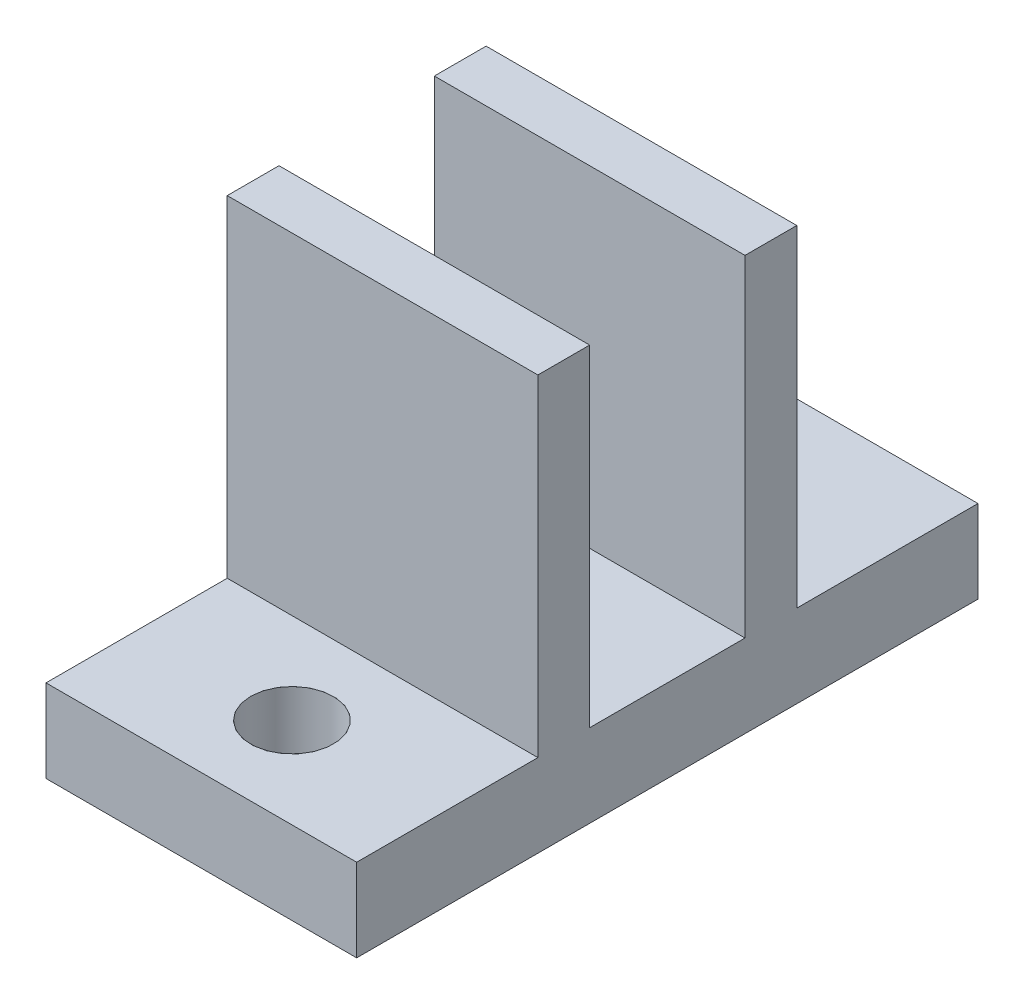
# Autodesk Inventor part: XPulleySupport
Saved by Autodesk Inventor 2019 (Build 230136000, 136)
## iProperties
Created: 2019-08-19
Part Number: XPulleySupport
Material: Generic
Document SubType Name: Modeling
Designer: Bruno
Density: 1 g/cm^3
Appearance: Default
Author: Bruno
Autodesk Inventor part; units mm, degrees
ref_plane "YZ Plane" through (0, 0, 0) normal (1, 0, 0) x (0, 1, 0)
ref_plane "XZ Plane" through (0, 0, 0) normal (0, 1, 0) x (-1, 0, 0)
ref_plane "XY Plane" through (0, 0, 0) normal (0, 0, 1) x (1, 0, 0)
sketch "Sketch1" plane through (0, 0, 0) normal (0, 1, 0) x (-1, 0, 0)
  line L0 (42.7623, -5.5692) -> (12.7623, -5.5692)
  line L1 (12.7623, 54.4308) -> (42.7623, 54.4308)
  line L2 (42.7623, 31.9308) -> (12.7623, 31.9308)
  line L3 (12.7623, 16.9308) -> (42.7623, 16.9308)
  line L4 (42.7623, 16.9308) -> (42.7623, 11.9308)
  line L5 (42.7623, 11.9308) -> (12.7623, 11.9308)
  line L6 (12.7623, 11.9308) -> (12.7623, 16.9308)
  line L7 (42.7623, 31.9308) -> (42.7623, 36.9308)
  line L8 (42.7623, 36.9308) -> (12.7623, 36.9308)
  line L9 (12.7623, 36.9308) -> (12.7623, 31.9308)
  line L10 (42.7623, 11.9308) -> (42.7623, -5.5692)
  line L11 (12.7623, 11.9308) -> (12.7623, -5.5692)
  line L12 (12.7623, 16.9308) -> (12.7623, 31.9308)
  line L13 (42.7623, 31.9308) -> (42.7623, 16.9308)
  line L14 (42.7623, 36.9308) -> (42.7623, 54.4308)
  line L15 (12.7623, 54.4308) -> (12.7623, 36.9308)
  circle A0 centre (27.7623, 3.1808) radius 4
  circle A1 centre (27.7623, 45.6808) radius 4
  line L16 (27.7623, 3.1808) -> (42.7623, 3.1808) construction
  line L17 (27.7623, 3.1808) -> (27.7623, 11.9308) construction
  line L18 (27.7623, 45.6808) -> (27.7623, 36.9308) construction
  line L19 (27.7623, 45.6808) -> (42.7623, 45.6808) construction
  point P0 (0, 0)
  dimension "d0" = 60
  dimension "d1" = 30
  dimension "d2" = 5
  dimension "d3" = 15
  dimension "d4" = 8
  dimension "d5" = 8
  constraints: 40 end point, 5 equal length, 5 perpendicular, 4 midpoint, 4 parallel, 2 centre point, 2 collinear, 1 horizontal, 1 vertical, 4 other
  measures "d0" distance of L0.end L1.start
  measures "d1" distance of L0.start L0.end
  measures "d2" distance of L9.start L12.end
  measures "d3" distance of L3.start L12.end
  measures "d4" diameter of A0
  measures "d5" diameter of A1
extrude "Extrusion1" add sketch "Sketch1" along normal blind 8 contours L0 L11 L5 L10 | L3 L12 L2 L13 | L8 L15 L1 L14
extrude "Extrusion2" add sketch "Sketch1" along normal blind 40 contours L5 L6 L3 L4 | L2 L9 L8 L7
body "Solid1"
